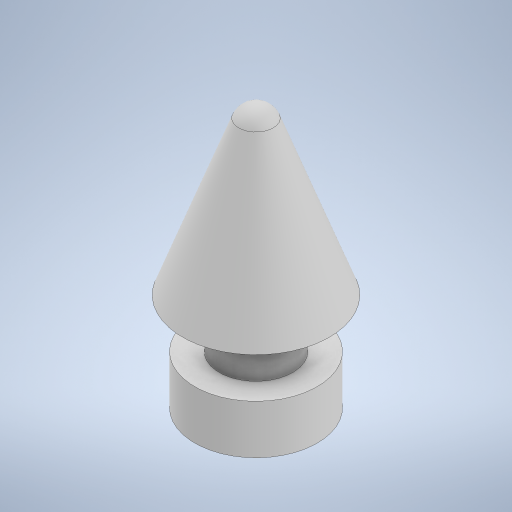
# Autodesk Inventor part: apple pensil tip
Saved by Autodesk Inventor 2024.3 (Build 283343000, 343)
## iProperties
Created: 2024-08-06
Part Number: apple pensil tip
Material: 일반
Document SubType Name: Modeling
Designer: naru4
Density: 1 g/cm^3
Appearance: 기본값
Author: naru4
Autodesk Inventor part; units mm, degrees
ref_plane "YZ Plane" through (0, 0, 0) normal (1, 0, 0) x (0, 1, 0)
ref_plane "XZ Plane" through (0, 0, 0) normal (0, 1, 0) x (-1, 0, 0)
ref_plane "XY Plane" through (0, 0, 0) normal (0, 0, 1) x (1, 0, 0)
sketch "스케치1" plane through (0, 0, 0) normal (1, 0, 0) x (0, 1, 0)
  line L0 (0, -1.5) -> (0, -3)
  arc A0 (6.2583, -0.7041) -> (6.75, 0) centre (6, 0) ccw
  line L1 (0, -3) -> (6.2583, -0.7041)
  line L2 (6.75, 0) -> (0, 0)
  line L3 (0, -1.5) -> (-2, -1.5)
  line L4 (-2, -1.5) -> (-2, -2.5)
  line L5 (-2, -2.5) -> (-4, -2.5)
  line L6 (-4, -2.5) -> (-4, 0)
  line L7 (-4, 0) -> (0, 0)
  dimension "d0" = 3
  dimension "d2" = 1.5
  dimension "d3" = 2
  dimension "d4" = 1
  dimension "d5" = 2
  constraints: 16 end point, 5 perpendicular, 2 point on circle, 1 centre point, 1 horizontal, 1 tangent, 1 vertical
  measures "d0" distance of L2.end L0.end
  measures "d2" diameter of A0
  measures "d3" distance of L0.start L3.end
  measures "d4" distance of L3.end L4.end
  measures "d5" distance of L4.end L5.end
revolve "회전1" add sketch "스케치1" angle 360 about axis through (0, 6.75, 0) along (0, -1, 0)
sketch "스케치2" plane through (0, -4, 0) normal (0, -1, 0) x (1, 0, 0)
  circle A0 centre (0, 0) radius 2
  dimension "d7" = 4
  constraints: 1 centre point, 1 coincident
  measures "d7" diameter of A0
extrude "돌출1" cut sketch "스케치2" against normal blind 1
